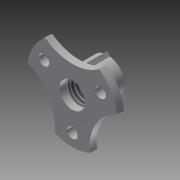
# Autodesk Inventor part: 5_16_18_tee_nut
Saved by Autodesk Inventor 2014 (Build 180170000, 170)
## iProperties
Created: 2015-03-07
Part Number: 5_16_18_tee_nut
Material: Generic
Document SubType Name: Modeling
Designer: cruiser
Density: 1 g/cm^3
Appearance: Steel
Author: cruiser
Autodesk Inventor part; units mm, degrees
ref_plane "YZ Plane" through (0, 0, 0) normal (1, 0, 0) x (0, 1, 0)
ref_plane "XZ Plane" through (0, 0, 0) normal (0, 1, 0) x (-1, 0, 0)
ref_plane "XY Plane" through (0, 0, 0) normal (0, 0, 1) x (1, 0, 0)
sketch "Sketch1" plane through (0, 0, 0) normal (0, 1, 0) x (-1, 0, 0)
  circle A0 centre (0, 0) radius 15.875
  dimension "d0" = 31.75
  constraints: 1 centre point, 1 coincident
  measures "d0" diameter of A0
extrude "Extrusion1" add sketch "Sketch1" along normal blind 2.4892
sketch "Sketch2" plane through (0, 2.4892, 0) normal (0, 1, 0) x (1, 0, 0)
  circle A0 centre (0, 0) radius 15.875 projected
  circle A1 centre (0, 11.5062) radius 1.8542
  line L0 (0, 0) -> (0, 15.875)
  circle A2 centre (-9.9647, -5.7531) radius 1.8542
  circle A3 centre (9.9647, -5.7531) radius 1.8542
  circle A4 centre (0, -25.4) radius 15.875
  line L1 (0, 0) -> (0, -25.4)
  circle A5 centre (21.997, 12.7) radius 15.875
  circle A6 centre (-21.997, 12.7) radius 15.875
  dimension "d3" = 3.7084
  dimension "d4" = 11.5062
  dimension "d7" = 360
  dimension "d9" = 31.75
  dimension "d10" = 25.4
  dimension "d13" = 360
  constraints: 6 centre point, 4 end point, 1 collinear, 1 point on line, 1 vertical, 1 vertical alignment, 15 other
  measures "d3" diameter of A1
  measures "d4" distance of L0.start A1.centre
  measures "d9" diameter of A4
  measures "d10" distance of L0.start L1.end
extrude "Extrusion2" cut sketch "Sketch2" against normal through all contours A0 A5 | A0 A5 | A4 A0 | A0 L1 A4 | A6 A0 | A0 A6 | A0 A4 L1
sketch "Sketch6" plane through (0, 2.4892, 0) normal (0, 1, 0) x (1, 0, 0)
  arc A0 (-15.761, -1.8989) -> (-9.525, -12.7) centre (0, 0) ccw projected
  arc A1 (6.236, 14.5989) -> (-6.236, 14.5989) centre (0, 0) ccw projected
  line L0 (0, 0) -> (0, 11.5062)
  circle A2 centre (0, 11.5062) radius 1.8542
  circle A3 centre (-9.9647, -5.7531) radius 1.8542
  circle A4 centre (9.9647, -5.7531) radius 1.8542
  arc A5 (9.525, -12.7) -> (15.761, -1.8989) centre (0, 0) ccw projected
  circle A6 centre (0, 0) radius 4.5
  dimension "d26" = 11.5062
  dimension "d27" = 3.7084
  dimension "d30" = 360
  dimension "d34" = 9
  constraints: 4 centre point, 2 coincident, 2 end point, 1 vertical, 7 other
  measures "d26" distance of L0.start L0.end
  measures "d27" diameter of A2
  measures "d34" diameter of A6
extrude "Extrusion5" cut sketch "Sketch6" against normal through all
sketch "Sketch3" plane through (0, 2.4892, 0) normal (0, 1, 0) x (1, 0, 0)
  arc A0 (9.525, -12.7) -> (15.761, -1.8989) centre (0, 0) ccw projected
  circle A1 centre (0, 0) radius 5.9944
  line L0 (0, -7.3323) -> (-6.35, 3.6662)
  line L1 (-6.35, 3.6662) -> (6.35, 3.6662)
  line L2 (6.35, 3.6662) -> (0, -7.3323)
  line L3 (0, 0) -> (0, -8.4562)
  dimension "d17" = 11.9888
  dimension "d18" = 12.7
  constraints: 8 end point, 2 coincident, 1 centre point, 1 point on line, 1 vertical, 7 other
  measures "d17" diameter of A1
  measures "d18" distance of L1.end L0.start
extrude "Extrusion3" add sketch "Sketch3" along normal blind 10.0076
sketch "Sketch4" plane through (0, 12.4968, 0) normal (0, 1, 0) x (1, 0, 0)
  arc A0 (-5.5463, 2.2741) -> (-0.8037, -5.9403) centre (0, 0) ccw projected
  circle A1 centre (0, 0) radius 3.9687
  dimension "d21" = 7.9375
  constraints: 1 centre point, 1 coincident
  measures "d21" diameter of A1
extrude "Extrusion4" cut sketch "Sketch4" against normal through all
thread "Thread1" size "5/16-18 UNC" class "2B" standard "ANSI Unified Screw Threads" full length
body "Solid1"
